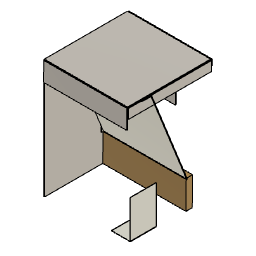
塗装ブース v8 (Autodesk Fusion 360 design; units mm, degrees)
Autodesk Fusion 360 part; units mm, degrees
note: some values were not read from the file. Set by a fixed rule: which face or edge a step refers to.
sketch "スケッチ1" plane through (0, 0, 0) normal (0, 1, 0) x (1, 0, 0) in component "塗装ブース"
  line L0 (0, 0) -> (350, 0)
  line L1 (350, 0) -> (350, -500)
  line L2 (350, -500) -> (0, -500)
  line L3 (0, -500) -> (0, 0)
  line L4 (340, -470) -> (150, -470)
  line L5 (150, -470) -> (150, -280)
  line L6 (150, -280) -> (340, -280)
  line L7 (340, -280) -> (340, -470)
  line L8 (315, -470) -> (315, -500) construction
  line L9 (350, -434.8785) -> (340, -434.8785)
  dimension "d1" = 350
  dimension "d2" = 500
  dimension "d3" = 190
  dimension "d4" = 190
  dimension "d5" = 30
  dimension "d6" = 10
  constraint horizontal L0
  constraint vertical L1
  constraint horizontal L2
  constraint vertical L3
  constraint coincident L0.start L3.end
  constraint horizontal L4
  constraint vertical L5
  constraint horizontal L6
  constraint vertical L7
  constraint coincident L4 L8.start
  constraint coincident L2 L8.end
  constraint perpendicular L2 L8
  constraint coincident L1 L9.start
  constraint coincident L7 L9.end
  constraint perpendicular L7 L9
  measures "d1" distance of L0.start L0.end
  measures "d2" distance of L0.start L2.end
  measures "d3" distance of L4.start L4.end
  measures "d4" distance of L4.start L6.end
  measures "d5" distance of L8.start L8.end
  measures "d6" distance of L9.start L9.end
sketch "スケッチ2" plane through (0, 0, 0) normal (1, 0, 0) x (0, 1, 0) in component "塗装ブース"
  line L0 (0, 0) -> (-350, 0)
  line L1 (-350, 0) -> (-350, 500)
  line L2 (-350, 500) -> (0, 500)
  line L3 (0, 500) -> (0, 0)
  line L4 (0, 500) -> (0, 475)
  line L5 (-205.9711, 100.0797) -> (-180.9711, 100.0797)
  line L6 (-180.9711, 100.0797) -> (-180.9711, 0.0797)
  line L7 (-180.9711, 0.0797) -> (-205.9711, 0.0797)
  line L8 (-205.9711, 0.0797) -> (-205.9711, 100.0797)
  circle A0 centre (0, 475) radius 425 construction
  line L9 (0, 475) -> (-246.3716, 128.6966)
  line L10 (0, 475) -> (-2.4445, 476.7391)
  line L11 (-2.4445, 476.7391) -> (-248.8099, 130.4443)
  line L12 (-246.3716, 128.6966) -> (-248.8099, 130.4443)
  dimension "d7" = 350
  dimension "d8" = 500
  dimension "d9" = 25
  dimension "d10" = 25
  dimension "d11" = 100
  dimension "d12" = 850
  dimension "d13" = 425
  dimension "d14" = 3
  constraint horizontal L0
  constraint vertical L1
  constraint horizontal L2
  constraint vertical L3
  constraint coincident L0.start L3.end
  constraint perpendicular L2 L4
  constraint horizontal L5
  constraint vertical L6
  constraint horizontal L7
  constraint vertical L8
  constraint coincident L4.end A0.centre
  constraint coincident A0 L9.end
  constraint perpendicular L9 L10
  constraint coincident A0 L11.end
  constraint perpendicular L10 L11
  measures "d7" distance of L0.start L0.end
  measures "d8" distance of L0.start L2.end
  measures "d9" distance of L2.end L4.end
  measures "d10" distance of L5.start L5.end
  measures "d11" distance of L5.start L7.end
  measures "d12" diameter of A0
  measures "d13" distance of L4.end L9.end
  measures "d14" distance of L4.end L10.end
extrude "押し出し1" add sketch "スケッチ1" against normal blind 3 makes body 1 in component "塗装ブース"
extrude "押し出し2" add sketch "スケッチ2" along normal blind 3 separate body contours L9 L10 L11 L12 | L0 L1 L2 L3 L4 | L5 L6 L7 L8 makes body 2 in component "塗装ブース"
ref_plane "作業平面1" through (175, -175, 250) normal (-1, 0, 0) x (0, -1, 0) in component "塗装ブース"
mirror "ミラー1" about plane through (175, -175, 250) normal (-1, 0, 0) of bodies 2 makes body 3 in component "塗装ブース"
sketch "スケッチ3" plane through (0, 0, 0) normal (0, 0, 1) x (1, 0, 0) in component "塗装ブース"
  line L0 (0, 0) -> (350, 0)
  line L1 (350, 0) -> (350, -350)
  line L2 (350, -350) -> (0, -350)
  line L3 (0, -350) -> (0, 0)
  dimension "d22" = 350
  dimension "d23" = 350
  constraint horizontal L0
  constraint vertical L1
  constraint horizontal L2
  constraint vertical L3
  constraint coincident L0.start L3.end
  measures "d22" distance of L0.start L0.end
  measures "d23" distance of L0.start L2.end
extrude "押し出し3" add sketch "スケッチ3" along normal blind 3 separate body makes body 4 in component "塗装ブース"
extrude "押し出し4" add sketch "スケッチ2" along normal blind 350 separate body contours L9 L10 L11 L12 makes body 5 in component "塗装ブース"
extrude "押し出し5" add sketch "スケッチ2" along normal blind 350 separate body contours L5 L6 L7 L8 makes body 6 in component "塗装ブース"
move_body "移動1" bodies 5 to x (1, 0, 0) y (0, 0.992546, 0.121869) z (0, -0.121869, 0.992546) at (0, 58.0817, 3.8514) in component "塗装ブース"
move_face "面を移動1" by (5, 0, 0) 1 faces at (0, -135.5716, 226.6252) on bodies 5 in component "塗装ブース"
move_face "面を移動2" by (-5, 0, 0) 1 faces at (350, -135.5716, 226.6252) on bodies 5 in component "塗装ブース"
copy_body "ボディのコピーと貼り付け1" bodies 4 makes body 7 in component "塗装ブース"
move_body "移動2" bodies 7 to x (1, 0, 0) y (0, 1, 0) z (0, 0, 1) at (0, 0, 500) in component "塗装ブース"
sketch "スケッチ4" plane through (3, 0, 0) normal (1, 0, 0) x (0, 1, 0) in component "塗装ブース"
  line L0 (0, 500) -> (-350, 500)
  line L1 (-350, 500) -> (-350, 0)
  line L2 (-350, 0) -> (0, 0)
  line L3 (0, 0) -> (0, 500)
  line L4 (0, 200) -> (-100, 0)
  line L5 (-100, 0) -> (-102.6833, 1.3416)
  line L6 (0, 200) -> (-2.6833, 201.3416)
  line L7 (-2.6833, 201.3416) -> (-102.6833, 1.3416)
  dimension "d30" = 3
  dimension "d31" = 3
  constraint coincident L3 L4.start
  constraint coincident L2 L4.end
  constraint perpendicular L4 L5
  constraint perpendicular L4 L6
  measures "d30" distance of L4.end L5.end
  measures "d31" distance of L4.start L6.end
extrude "押し出し6" add sketch "スケッチ4" along normal blind 340 separate body contours L4 L5 L6 L7 makes body 8 in component "塗装ブース"
move_body "移動3" bodies 8 to x (1, 0, 0) y (0, 1, 0) z (0, 0, 1) at (0, 0, 75) in component "塗装ブース"
move_face "面を移動3" by (0, -36.6715, -73.343) 1 faces at (116.3333, -100.8944, 75.4472) on bodies 8 in component "塗装ブース"
move_face "面を移動4" by (0, -40.2492, -80.4984) 1 faces at (229.6667, -1.7889, 275.8944) on bodies 8 in component "塗装ブース"
move_body "移動4" bodies 8 to x (1, 0, 0) y (0, 1, 0) z (0, 0, 1) at (0, 41, 0) in component "塗装ブース"
move_body "移動5" bodies 5 to x (1, 0, 0) y (0, 0.642788, 0.766044) z (0, -0.766044, 0.642788) at (0, 5.7568, 193.6568) in component "塗装ブース"
move_body "移動6" bodies 5 to x (1, 0, 0) y (0, 1, 0) z (0, 0, 1) at (0, 100, 0) in component "塗装ブース"
move_body "移動7" bodies 6 to x (1, 0, 0) y (0, 1, 0) z (0, 0, 1) at (0, 100, 0) in component "塗装ブース"
move_body "移動8" bodies 5 to x (1, 0, 0) y (0, 0.984808, 0.173648) z (0, -0.173648, 0.984808) at (0, 16.2943, 19.7581) in component "塗装ブース"
move_body "移動9" bodies 5 to x (1, 0, 0) y (0, 0.996195, -0.087156) z (0, 0.087156, 0.996195) at (0, -2.7934, -12.609) in component "塗装ブース"
move_face "面を移動5" by (0, 26.8381, -53.663) 1 faces at (118.3333, -286.4983, 480.1295) on bodies 5 in component "塗装ブース"
copy_body "ボディのコピーと貼り付け2" bodies 5 makes body 9 in component "塗装ブース"
move_body "移動10" bodies 9 to x (1, 0, 0) y (0, 0.891007, -0.45399) z (0, 0.45399, 0.891007) at (0, -231.01, -96.0407) in component "塗装ブース"
move_face "面を移動6" by (0, -2.0979, -279.9921) 1 faces at (118.3333, -268.7571, 401.827) on bodies 9 in component "塗装ブース"
move_body "移動11" bodies 9 to x (1, 0, 0) y (0, 1, 0) z (0, 0, 1) at (0, -25.6328, 378.6324) in component "塗装ブース"
move_face "面を移動7" by (0, -0.2755, -24.9985) 1 faces at (118.3333, -297.1247, 415.4732) on bodies 9 in component "塗装ブース"
copy_body "ボディのコピーと貼り付け3" bodies 6 makes body 10 in component "塗装ブース"
move_body "移動12" bodies 10 to x (1, 0, 0) y (0, 1, 0) z (0, 0, 1) at (0, 60, 0) in component "塗装ブース"
move_body "位置合わせ1" bodies 10 to x (1, 0, 0) y (0, 0.894383, 0.447302) z (0, -0.447302, 0.894383) at (0, 0.4446, 11.3952) in component "塗装ブース"
move_body "移動13" bodies 10 to x (1, 0, 0) y (0, 1, 0) z (0, 0, 1) at (0, -8.946, 17.8877) in component "塗装ブース"
copy_body "ボディのコピーと貼り付け4" bodies 10 makes body 11 in component "塗装ブース"
move_body "移動14" bodies 11 to x (1, 0, 0) y (0, 1, 0) z (0, 0, 1) at (0, -190.1033, 380.1128) in component "塗装ブース"
move_face "面を移動8" by (0, 17.8921, -35.7753) 1 faces at (118.3333, -259.6601, 426.4665) on bodies 5 in component "塗装ブース"
copy_body "ボディ -> コンポーネント1" bodies 5 removing the originals makes body 12 in component "中板1"
copy_body "CutPasteBodies1" bodies 11 10 removing the originals makes body 13 makes body 14 in component "中板1"
move_body "移動1'" bodies 13 to x (1, 0, 0) y (0, 1, 0) z (0, 0, 1) at (0, -4.473, 8.9438) in component "中板1"
move_face "面を移動1'" by (0, -6.2622, 12.5214) 1 faces at (118.3333, -241.7681, 390.6912) on bodies 12 in component "中板1"
copy_body "CutPasteBodies5" bodies 13 14 removing the originals makes body 15 makes body 16 in component "塗装ブース"
move_body "移動15" bodies 16 to x (1, 0, 0) y (0, 0.891007, -0.45399) z (0, 0.45399, 0.891007) at (0, -55.0194, -27.1445) in component "塗装ブース"
move_body "移動16" bodies 15 to x (1, 0, 0) y (0, 0.898794, -0.438371) z (0, 0.438371, 0.898794) at (0, -245.4958, -66.4217) in component "塗装ブース"
move_body "移動17" bodies 15 to x (1, 0, 0) y (0, 1, 0) z (0, 0, 1) at (0, 49.9975, 0.498) in component "塗装ブース"
move_body "移動18" bodies 16 to x (1, 0, 0) y (0, 1, 0) z (0, 0, 1) at (0, -29.9992, 0.2248) in component "塗装ブース"
move_body "移動2'" bodies 12 to x (1, 0, 0) y (0, 0.996195, -0.087156) z (0, 0.087156, 0.996195) at (0, -36.015, -20.2422) in component "中板1"
move_face "面を移動2'" by (0, -4.3724, 11.1751) 1 faces at (118.3333, -123.3274, 87.7986) on bodies 12 in component "中板1"
move_face "面を移動9" by (0, 0.5511, 49.997) 1 faces at (118.3333, -297.312, 390.4737) on bodies 9 in component "塗装ブース"
move_face "面を移動3'" by (0, -11.0295, 27.8989) 1 faces at (118.3333, -247.9591, 403.0533) on bodies 12 in component "中板1"
move_body "移動3'" bodies 12 to x (1, 0, 0) y (0, 0.996195, -0.087156) z (0, 0.087156, 0.996195) at (0, -9.0544, -10.9217) in component "中板1"
move_body "移動19" bodies 9 to x (1, 0, 0) y (0, 1, 0) z (0, 0, 1) at (0, 39.9989, -0.2997) in component "塗装ブース"
move_body "移動4'" bodies 12 to x (1, 0, 0) y (0, 1, 0) z (0, 0, 1) at (0, -2.852, 9.5847) in component "中板1"
move_body "移動20" bodies 9 to x (1, 0, 0) y (0, 1, 0) z (0, 0, 1) at (0, -19.9994, 0.1498) in component "塗装ブース"
move_face "面を移動4'" by (0, 2.8181, -9.5947) 1 faces at (118.3333, -130.5347, 108.3778) on bodies 12 in component "中板1"
move_body "移動5'" bodies 12 to x (1, 0, 0) y (0, 0.996195, 0.087156) z (0, -0.087156, 0.996195) at (0, 8.0681, 11.6693) in component "中板1"
move_body "移動21" bodies 9 to x (1, 0, 0) y (0, 1, 0) z (0, 0, 1) at (0, -73.9979, 0.5544) in component "塗装ブース"
move_face "面を移動5'" by (0, -7.353, 18.5993) 1 faces at (118.3333, -262.6651, 440.2519) on bodies 12 in component "中板1"
move_face "面を移動10" by (0, -0.2204, -19.9988) 1 faces at (118.3333, -350.9359, 440.8772) on bodies 9 in component "塗装ブース"
sketch "スケッチ5" plane through (3, 0, 0) normal (1, 0, 0) x (0, 1, 0) in component "塗装ブース"
  line L0 (0, 500) -> (-350, 500)
  line L1 (-350, 500) -> (-350, 0)
  line L2 (-350, 0) -> (0, 0)
  line L3 (0, 0) -> (0, 500)
  line L4 (-350, 500) -> (-240, 500)
  line L5 (-240, 500) -> (-240, 460)
  line L6 (-240, 460) -> (-350, 460)
  line L7 (-350, 460) -> (-350, 500)
  line L8 (-350, 0) -> (-100, 0)
  line L9 (-100, 0) -> (-100, 120)
  line L10 (-100, 120) -> (-350, 120)
  line L11 (-350, 120) -> (-350, 0)
  line L12 (-100, 120) -> (-73, 120)
  line L13 (-73, 120) -> (-73, 0)
  line L14 (-73, 0) -> (-100, 0)
  line L15 (-100, 0) -> (-100, 120)
  line L16 (-240, 460) -> (-99.0891, 105.2934)
  line L17 (-99.0891, 105.2934) -> (-96.3011, 106.4009)
  line L18 (-240, 460) -> (-237.2119, 461.1076)
  line L19 (-237.2119, 461.1076) -> (-96.3011, 106.4009)
  dimension "d46" = 250
  dimension "d47" = 120
  dimension "d48" = 40
  dimension "d49" = 110
  dimension "d50" = 27
  dimension "d51" = 120
  dimension "d52" = 3
  dimension "d53" = 3
  constraint horizontal L4
  constraint vertical L5
  constraint horizontal L6
  constraint vertical L7
  constraint coincident L0.end L1.start
  constraint horizontal L8
  constraint vertical L9
  constraint horizontal L10
  constraint vertical L11
  constraint coincident L1.end L2.start
  constraint horizontal L12
  constraint vertical L13
  constraint horizontal L14
  constraint vertical L15
  constraint perpendicular L16 L17
  constraint perpendicular L16 L18
  constraint perpendicular L17 L19
  measures "d46" distance of L1.end L8.end
  measures "d47" distance of L1.end L10.end
  measures "d48" distance of L4.end L5.end
  measures "d49" distance of L5.end L6.end
  measures "d50" distance of L9.end L12.end
  measures "d51" distance of L9.end L8.end
  measures "d52" distance of L16.end L17.end
  measures "d53" distance of L5.end L18.end
extrude "押し出し7" add sketch "スケッチ5" along normal blind 340 separate body contours L10 L16 L18 L19 makes body 17 in component "塗装ブース"
move_face "面を移動11" by (0, 1.9999, -0.015) 1 faces at (116.6667, -99.7697, 69.9327) on bodies 16 in component "塗装ブース"
move_face "面を移動12" by (0, 0.1498, 19.9994) 1 faces at (116.6667, -115.5195, 103.385) on bodies 16 in component "塗装ブース"
move_body "移動22" bodies 16 to x (1, 0, 0) y (0, 1, 0) z (0, 0, 1) at (0, -8.7841, -3.4099) in component "塗装ブース"
move_body "移動23" bodies 16 to x (1, 0, 0) y (0, 1, 0) z (0, 0, 1) at (0, 29.9992, -0.2248) in component "塗装ブース"
copy_body "ボディのコピーと貼り付け6" bodies 9 makes body 18 in component "塗装ブース"
move_body "移動24" bodies 18 to x (1, 0, 0) y (0, 1, 0) z (0, 0, 1) at (0, 249.993, -1.8731) in component "塗装ブース"
sketch "スケッチ6" plane through (3, 0, 0) normal (1, 0, 0) x (0, 1, 0) in component "塗装ブース"
  circle A0 centre (-110, 130) radius 4
  line L0 (-350, 0) -> (-110, 0)
  line L1 (-110, 0) -> (-110, 130)
  line L2 (-110, 130) -> (-350, 130)
  line L3 (-350, 130) -> (-350, 0)
  line L4 (-350, 500) -> (-245, 500)
  line L5 (-245, 500) -> (-245, 464)
  line L6 (-245, 460) -> (-350, 460)
  line L7 (-350, 460) -> (-350, 500)
  line L8 (-246.9279, 456.4953) -> (-248.453, 453.7226)
  line L9 (-241.5481, 462.0211) -> (-238.8174, 463.6199)
  line L10 (-231.7545, 450.441) -> (-229.1103, 451.8581)
  line L11 (-229.1103, 451.8581) -> (-236.9376, 466.4634)
  line L12 (-236.9376, 466.4634) -> (-244.3537, 467.1352)
  line L13 (-237.1247, 460.4616) -> (-239.7689, 459.0445)
  line L14 (-239.7689, 459.0445) -> (-234.451, 449.1215)
  line L15 (-234.451, 449.1215) -> (-237.0952, 447.7044)
  line L16 (-237.0952, 447.7044) -> (-240.6869, 454.4064)
  line L17 (-240.6869, 454.4064) -> (-239.7689, 459.0445)
  line L18 (-239.7689, 459.0445) -> (-241.5665, 462.0521)
  arc A1 (-241.5481, 462.0211) -> (-246.9279, 456.4953) centre (-245, 460) ccw
  line L19 (-238.8174, 463.6199) -> (-238.5621, 463.1437)
  line L20 (-237.1247, 460.4616) -> (-231.7545, 450.441)
  arc A2 (-238.5621, 463.1437) -> (-238.8174, 463.6199) centre (-245, 460) ccw
  arc A3 (-244.3537, 467.1352) -> (-248.453, 453.7226) centre (-245, 460) ccw
  circle A4 centre (-245, 460) radius 4
  dimension "d57" = 8
  dimension "d58" = 240
  dimension "d59" = 130
  dimension "d60" = 8
  dimension "d61" = 105
  dimension "d62" = 40
  dimension "d63" = 3
  dimension "d64" = 3
  dimension "d65" = 3
  dimension "d66" = 8
  constraint horizontal L0
  constraint vertical L1
  constraint horizontal L2
  constraint vertical L3
  constraint coincident A0.centre L1.end
  constraint horizontal L4
  constraint vertical L5
  constraint horizontal L6
  constraint vertical L7
  constraint coincident L6.start A1.centre
  constraint concentric A1 A2
  constraint perpendicular L10 L19
  constraint perpendicular L10 L11
  constraint coincident L12.end A2
  constraint tangent L12 A2
  constraint coincident L13.start L19
  constraint perpendicular L13 L19
  constraint perpendicular L13 L14
  constraint perpendicular L14 L15
  constraint perpendicular L15 L16
  constraint coincident L18.end A1
  constraint tangent L18 A1
  constraint collinear L19 L20
  constraint concentric A2 A3
  constraint coincident A1 L5.end
  measures "d57" diameter of A0
  measures "d58" distance of L0.start L0.end
  measures "d59" distance of L0.start L2.end
  measures "d60" diameter of A1
  measures "d61" distance of L4.start L4.end
  measures "d62" distance of L4.end L6.start
  measures "d63" distance of L10.start L10.end
  measures "d64" distance of L13.start L13.end
  measures "d65" distance of L14.end L15.end
  measures "d66" diameter of A4
move_face "面を移動13" by (0, -0.5511, -49.997) 1 faces at (118.3333, -101.0927, 419.0045) on bodies 18 in component "塗装ブース"
move_body "移動25" bodies 18 to x (1, 0, 0) y (0, 1, 0) z (0, 0, 1) at (0, -24.9993, 0.1873) in component "塗装ブース"
extrude "押し出し1'" add sketch "スケッチ6" along normal blind 370 and the other way blind 20 separate body contours L18 A1 A4 makes body 19
copy_body "CutPasteBodies7" bodies 19 removing the originals makes body 20 in component "塗装ブース"
copy_body "ボディのコピーと貼り付け1'" bodies 20 makes body 21
move_body "移動1''" bodies 21 to x (1, 0, 0) y (0, 1, 0) z (0, 0, 1) at (0, 117.9673, -299.029)
copy_body "ボディのコピーと貼り付け2'" bodies 20 makes body 22
move_body "移動2''" bodies 22 to x (1, 0, 0) y (0, 1, 0) z (0, 0, 1) at (0, 112, -84)
move_body "移動26" bodies 20 to x (1, 0, 0) y (0, 1, 0) z (0, 0, 1) at (0, 0, 25) in component "塗装ブース"
move_body "移動27" bodies 20 to x (1, 0, 0) y (0, 1, 0) z (0, 0, 1) at (0, 0, -20) in component "塗装ブース"
move_body "移動3''" bodies 22 to x (1, 0, 0) y (0, 1, 0) z (0, 0, 1) at (0, 12, 13)
sketch "スケッチ1 (2)" plane through (3, 0, 0) normal (1, 0, 0) x (0, 1, 0)
  line L0 (-275, 0) -> (-165, 0)
  line L1 (-165, 0) -> (-165, 1)
  line L2 (-165, 1) -> (-275, 1)
  line L3 (-275, 1) -> (-275, 0)
  dimension "d83" = 110
  dimension "d84" = 1
  constraint horizontal L0
  constraint vertical L1
  constraint horizontal L2
  constraint vertical L3
  measures "d83" distance of L0.start L0.end
  measures "d84" distance of L0.start L2.end
extrude "押し出し2'" add sketch "スケッチ1 (2)" along normal blind 80 separate body makes body 23
sketch "スケッチ2 (2)" plane through (0, 0, 1) normal (0, 0, 1) x (-1, 0, 0)
  line L0 (-3, 165) -> (-3, 275)
  line L1 (-3, 275) -> (-83, 275)
  line L2 (-83, 275) -> (-83, 165)
  line L3 (-83, 165) -> (-3, 165)
  line L4 (-3, 165) -> (-4, 165)
  line L5 (-4, 165) -> (-4, 275)
  line L6 (-4, 275) -> (-3, 275)
  line L7 (-3, 275) -> (-3, 165)
  dimension "d87" = 1
  dimension "d88" = 110
  constraint horizontal L4
  constraint vertical L5
  constraint horizontal L6
  constraint vertical L7
  constraint coincident L0.start L3.end
  measures "d87" distance of L0.start L4.end
  measures "d88" distance of L0.start L0.end
extrude "押し出し3'" add sketch "スケッチ2 (2)" along normal blind 160 contours L0 L1 L3 L4 L5 L6 L7 bodies 23
move_body "移動4''" bodies 23 to x (1, 0, 0) y (0, 1, 0) z (0, 0, 1) at (10, 0, 10)
move_body "移動5''" bodies 23 to x (1, 0, 0) y (0, 1, 0) z (0, 0, 1) at (0, 0, -7)
move_body "移動6'" bodies 23 to x (1, 0, 0) y (0, 1, 0) z (0, 0, 1) at (-10, 0, 0)
move_body "移動7'" bodies 23 to x (1, 0, 0) y (0, 1, 0) z (0, 0, 1) at (0, 20, 0)
ref_plane "作業平面1" through (175, -175, 250) normal (-1, 0, 0) x (0, 0, -1)
mirror "ミラー1'" about plane through (175, -175, 250) normal (-1, 0, 0) of bodies 23 makes body 24
copy_body "CutPasteBodies8" bodies 21 22 23 24 removing the originals makes body 25 makes body 26 makes body 27 makes body 28 in component "塗装ブース"
delete_body "RemoveBody5" bodies 8 in component "塗装ブース"
delete_body "RemoveBody6" bodies 6 in component "塗装ブース"
move_body "移動28" bodies 18 26 to x (1, 0, 0) y (0, 1, 0) z (0, 0, 1) at (0, -20, 0) in component "塗装ブース"
move_body "移動29" bodies 27 28 to x (1, 0, 0) y (0, 1, 0) z (0, 0, 1) at (0, -80, 0) in component "塗装ブース"
copy_body "ボディのコピーと貼り付け1''" bodies 1 2 4 3 7 9 16 20 15 25 18 27 28 17 26 makes body 29 makes body 30 makes body 31 makes body 32 makes body 33 makes body 34 makes body 35 makes body 36 makes body 37 makes body 38 makes body 39 makes body 40 makes body 41 makes body 42 makes body 43 in component "塗装ブース2"
sketch "スケッチ1 (3)" plane through (0, 0, 3) normal (0, 0, 1) x (-1, 0, 0) in component "塗装ブース2"
  line L0 (0, 350) -> (-350, 350)
  line L1 (-350, 350) -> (-350, 0)
  line L2 (-350, 0) -> (0, 0)
  line L3 (0, 0) -> (0, 350)
  line L4 (-38.9588, 123.5058) -> (-158.9588, 123.5058)
  line L5 (-158.9588, 123.5058) -> (-158.9588, 150.5058)
  line L6 (-158.9588, 150.5058) -> (-38.9588, 150.5058)
  line L7 (-38.9588, 150.5058) -> (-38.9588, 123.5058)
  dimension "d111" = 120
  dimension "d112" = 27
  constraint horizontal L4
  constraint vertical L5
  constraint horizontal L6
  constraint vertical L7
  measures "d111" distance of L4.start L4.end
  measures "d112" distance of L4.start L6.end
extrude "押し出し1''" add sketch "スケッチ1 (3)" along normal blind 485 separate body contours L4 L5 L6 L7 makes body 44 in component "塗装ブース2"
copy_body "ボディのコピーと貼り付け2''" bodies 44 makes body 45 in component "塗装ブース2"
move_body "移動1'''" bodies 45 to x (1, 0, 0) y (0, 1, 0) z (0, 0, 1) at (120, 0, 0) in component "塗装ブース2"
move_body "移動2'''" bodies 44 45 to x (1, 0, 0) y (0, 1, 0) z (0, 0, 1) at (-35, 0, 0) in component "塗装ブース2"
delete_body "RemoveBody7" bodies 15 in component "塗装ブース"
move_face "面を移動14" by (0, -14.7678, 37.1741) 1 faces at (116.3333, -239.0706, 460.3692) on bodies 17 in component "塗装ブース"
sketch "スケッチ7" plane through (0, -49.4554, -19.6467) normal (0, -0.929352, -0.369195) x (1, 0, 0) in component "塗装ブース"
  line L0 (3, 556.1087) -> (3, 150.2624)
  line L1 (3, 150.2624) -> (343, 150.2624)
  line L2 (343, 150.2624) -> (343, 556.1087)
  line L3 (343, 556.1087) -> (3, 556.1087)
  line L4 (3, 556.1087) -> (18, 556.1087)
  line L5 (18, 556.1087) -> (18, 546.1087)
  line L6 (18, 546.1087) -> (3, 546.1087)
  line L7 (3, 546.1087) -> (3, 556.1087)
  line L8 (343, 556.1087) -> (328, 556.1087)
  line L9 (328, 556.1087) -> (328, 546.1087)
  line L10 (328, 546.1087) -> (343, 546.1087)
  line L11 (343, 546.1087) -> (343, 556.1087)
  line L12 (18, 546.1087) -> (328.5453, 546.1087)
  line L13 (328.5453, 546.1087) -> (328.5453, 506.1087)
  line L14 (328.5453, 506.1087) -> (18, 506.1087)
  line L15 (18, 506.1087) -> (18, 546.1087)
  dimension "d115" = 15
  dimension "d116" = 10
  dimension "d117" = 15
  dimension "d118" = 10
  dimension "d119" = 310.5453
  dimension "d120" = 40
  constraint horizontal L4
  constraint vertical L5
  constraint horizontal L6
  constraint vertical L7
  constraint coincident L0.start L3.end
  constraint horizontal L8
  constraint vertical L9
  constraint horizontal L10
  constraint vertical L11
  constraint coincident L2.end L3.start
  constraint horizontal L12
  constraint vertical L13
  constraint horizontal L14
  constraint vertical L15
  measures "d115" distance of L0.start L4.end
  measures "d116" distance of L0.start L6.end
  measures "d117" distance of L2.end L8.end
  measures "d118" distance of L2.end L10.end
  measures "d119" distance of L5.end L12.end
  measures "d120" distance of L5.end L14.end
extrude "押し出し8" cut sketch "スケッチ7" against normal blind 20 contours L10 L12 L13 L14 L15 bodies 17 in component "塗装ブース"
move_face "面を移動15" by (0, 0.4409, 39.9976) 1 faces at (118.3333, -146.4667, 369.193) on bodies 18 in component "塗装ブース"
copy_body "ボディのコピーと貼り付け9" bodies 9 makes body 46 in component "塗装ブース"
move_body "移動30" bodies 46 to x (1, 0, 0) y (0, 0, -1) z (0, 1, 0) at (0, -715.392, 145.3667) in component "塗装ブース"
move_face "面を移動16" by (0, -39.9989, 0.2997) 1 faces at (118.3333, -214.5202, 495.853) on bodies 46 in component "塗装ブース"
move_face "面を移動17" by (0, -3.6919, 9.2935) 1 faces at (225.0302, -235.3787, 451.0757) on bodies 17 in component "塗装ブース"
sketch "スケッチ8" plane through (3, 0, 0) normal (1, 0, 0) x (0, 1, 0) in component "塗装ブース"
extrude "押し出し9" add sketch "スケッチ5" along normal blind 340 contours L9 L10 L15 L16 L19 | L9 L15 L16 L17 L19 bodies 17 in component "塗装ブース"
move_face "面を移動18" by (10, 0, 0) 1 faces at (343, -149.1233, 236.6587) on bodies 17 in component "塗装ブース"
move_body "移動31" bodies 2 to x (1, 0, 0) y (0, 1, 0) z (0, 0, 1) at (-3, 0, 0) in component "塗装ブース"
move_body "移動32" bodies 3 to x (1, 0, 0) y (0, 1, 0) z (0, 0, 1) at (3, 0, 0) in component "塗装ブース"
move_body "移動33" bodies 1 to x (1, 0, 0) y (0, 1, 0) z (0, 0, 1) at (0, 3, 0) in component "塗装ブース"
move_body "移動34" bodies 4 to x (1, 0, 0) y (0, 1, 0) z (0, 0, 1) at (0, 0, -3) in component "塗装ブース"
move_body "移動35" bodies 9 to x (1, 0, 0) y (0, 1, 0) z (0, 0, 1) at (-5.0412, 3.6759, -1.0303) in component "塗装ブース"
move_face "面を移動19" by (10, 0, 0) 1 faces at (339.9588, -347.21, 446.5132) on bodies 9 in component "塗装ブース"
move_body "移動36" bodies 9 to x (1, 0, 0) y (0, 1, 0) z (0, 0, 1) at (0, -3.9999, 0.03) in component "塗装ブース"
move_face "面を移動20" by (0, 28.9186, -72.7952) 1 faces at (119.6667, -98.1598, 105.6625) on bodies 17 in component "塗装ブース"
move_face "面を移動21" by (0, -33.2275, 83.6417) 1 faces at (119.6667, -69.2411, 32.8673) on bodies 17 in component "塗装ブース"
move_body "移動37" bodies 46 to x (1, 0, 0) y (0, 1, 0) z (0, 0, 1) at (-2, 0, 0) in component "塗装ブース"
move_face "面を移動22" by (10, 0, 0) 1 faces at (343, -281.1814, 496.3525) on bodies 46 in component "塗装ブース"
move_face "面を移動23" by (9.455, 0, 0) 1 faces at (328.5453, -246.4545, 478.9562) on bodies 17 in component "塗装ブース"
move_face "面を移動24" by (10, 0, 0) 1 faces at (345, -145.9422, 439.1912) on bodies 18 in component "塗装ブース"
copy_body "CutPasteBodies1'" bodies 2 7 9 18 removing the originals makes body 47 makes body 48 makes body 49 makes body 50 in component "001"
copy_body "CutPasteBodies1''" bodies 1 4 3 removing the originals makes body 51 makes body 52 makes body 53 in component "002"
move_body "移動1''''" bodies 50 to x (1, 0, 0) y (0, 1, 0) z (0, 0, 1) at (-5, 0, 0) in component "001"
copy_body "CutPasteBodies1'''" bodies 46 17 removing the originals makes body 54 makes body 55 in component "003"
delete_body "RemoveBody17" bodies 17 in component "塗装ブース"
delete_body "RemoveBody18" bodies 46 in component "塗装ブース"
sketch "スケッチ9" plane through (0, 0, 0) normal (1, 0, 0) x (0, 1, 0) in component "塗装ブース"
  line L0 (0, 500) -> (-350, 500)
  line L1 (-350, 500) -> (-350, 0)
  line L2 (-350, 0) -> (0, 0)
  line L3 (0, 0) -> (0, 500)
  line L4 (-90, 110) -> (-106, 110)
  line L5 (-106, 110) -> (-106, 182)
  line L6 (-106, 182) -> (-90, 182)
  line L7 (-90, 182) -> (-90, 110)
  line L8 (-90, 110) -> (-106, 182) construction
  line L9 (-106, 110) -> (-90, 182) construction
  line L10 (0, 150) -> (-90, 150)
  line L11 (-90, 0) -> (-90, 110)
  point P0 (-98, 146)
  dimension "d125" = 16
  dimension "d126" = 72
  dimension "d127" = 90
  dimension "d128" = 110
  constraint horizontal L4
  constraint perpendicular L4 L5
  constraint parallel L4 L6
  constraint parallel L5 L7
  constraint coincident L8 P0
  constraint coincident L9 P0
  constraint coincident L3 L10.start
  constraint perpendicular L7 L10
  constraint coincident L2 L11.start
  constraint perpendicular L4 L11
  measures "d125" distance of L5.end L6.end
  measures "d126" distance of L4.end L5.end
  measures "d127" distance of L10.start L10.end
  measures "d128" distance of L11.start L4.start
extrude "押し出し10" add sketch "スケッチ9" along normal blind 2 separate body contours L4 L5 L6 L7 makes body 56 in component "塗装ブース"
copy_body "ボディのコピーと貼り付け10" bodies 50 makes body 57 in component "塗装ブース"
move_body "移動38" bodies 57 to x (1, 0, 0) y (0, 1, 0) z (0, 0, 1) at (0, 151.0107, 0.8686) in component "塗装ブース"
move_face "面を移動25" by (0, 0.5511, 49.997) 1 faces at (116.6667, 4.8438, 410.0607) on bodies 57 in component "塗装ブース"
copy_body "CutPasteBodies2" bodies 57 removing the originals makes body 58 in component "001"
copy_body "ボディのコピーと貼り付け2'''" bodies 52 makes body 59 in component "002"
move_body "移動1'''''" bodies 59 to x (1, 0, 0) y (0, 1, 0) z (0, 0, 1) at (-400, 0, 0) in component "002"
move_face "面を移動1''" by (310, 0, 0) 1 faces at (-400, -233.3333, -1) on bodies 59 in component "002"
move_body "移動2''''" bodies 59 to x (0, 0, -1) y (0, 1, 0) z (1, 0, 0) at (-2, 0, -53) in component "002"
copy_body "ボディのコピーと貼り付け3'" bodies 59 makes body 60 in component "001"
move_body "移動2'''''" bodies 60 to x (1, 0, 0) y (0, 1, 0) z (0, 0, 1) at (356, 0, 463) in component "001"
copy_body "ボディのコピーと貼り付け3''" bodies 51 makes body 61 in component "002"
move_body "移動3'''" bodies 61 to x (1, 0, 0) y (0, 1, 0) z (0, 0, 1) at (-425, 0, 0) in component "002"
move_face "面を移動2''" by (-310, 0, 0) 2 faces at (-75, 1, 144.9595) (-75, 2, 456.5857) on bodies 61 in component "002"
move_body "移動4'''" bodies 61 to x (1, 0, 0) y (0, 1, 0) z (0, 0, 1) at (380, 0, 0) in component "002"
move_body "移動5'''" bodies 61 to x (0, 1, 0) y (-1, 0, 0) z (0, 0, 1) at (-2, 8, 0) in component "002"
move_face "面を移動3''" by (0, -50, 0) 1 faces at (-4, 0, 23.6667) on bodies 59 in component "002"
copy_body "ボディのコピーと貼り付け11" bodies 52 makes body 62 in component "塗装ブース"
move_body "移動39" bodies 62 to x (1, 0, 0) y (0, 1, 0) z (0, 0, 1) at (0, 390, 0) in component "塗装ブース"
move_face "面を移動26" by (0, -310, 0) 1 faces at (116.6667, 390, -1) on bodies 62 in component "塗装ブース"
move_body "移動40" bodies 62 to x (1, 0, 0) y (0, 1, 0) z (0, 0, 1) at (0, -35, 0) in component "塗装ブース"
move_body "移動41" bodies 62 to x (1, 0, 0) y (0, 0, 1) z (0, -1, 0) at (0, 2, -8) in component "塗装ブース"
copy_body "CutPasteBodies4" bodies 62 removing the originals makes body 63 in component "002"
move_face "面を移動1'''" by (0, 0.1653, 14.9991) 1 faces at (116.6667, 5.2184, 460.0596) on bodies 58 in component "001"
move_body "移動42" bodies 56 to x (1, 0, 0) y (0, 0, 1) z (0, -1, 0) at (0, 40, 224) in component "塗装ブース"
move_body "移動43" bodies 56 to x (1, 0, 0) y (0, 1, 0) z (0, 0, 1) at (0, 20, 0) in component "塗装ブース"
copy_body "ボディのコピーと貼り付け12" bodies 56 makes body 64 in component "塗装ブース"
move_body "移動44" bodies 64 to x (1, 0, 0) y (0, 1, 0) z (0, 0, 1) at (350, 0, 0) in component "塗装ブース"
copy_body "CutPasteBodies5'" bodies 64 removing the originals makes body 65 in component "002"
copy_body "CutPasteBodies4'" bodies 56 removing the originals makes body 66 in component "001"
delete_body "RemoveBody23" bodies 20 in component "塗装ブース"
delete_body "RemoveBody24" bodies 25 in component "塗装ブース"
delete_body "RemoveBody25" bodies 26 in component "塗装ブース"
move_body "移動3''''" bodies 66 to x (1, 0, 0) y (0, 1, 0) z (0, 0, 1) at (0, 15, 0) in component "001"
move_body "移動6''" bodies 65 to x (1, 0, 0) y (0, 1, 0) z (0, 0, 1) at (0, 15, 0) in component "002"
move_body "移動7''" bodies 65 to x (1, 0, 0) y (0, 1, 0) z (0, 0, 1) at (0, -5, 0) in component "002"
move_body "移動4''''" bodies 66 to x (1, 0, 0) y (0, 1, 0) z (0, 0, 1) at (0, -5, 0) in component "001"
component "塗装ブース" placed x (1, 0, 0) y (0, 1, 0) z (0, 0, 1) at (0, 0, 0)
component "塗装ブース2" placed x (1, 0, 0) y (0, 1, 0) z (0, 0, 1) at (0, 0, 0)
component "001" placed x (1, 0, 0) y (0, 1, 0) z (0, 0, 1) at (0, 0, 0) in component "塗装ブース"
component "002" placed x (1, 0, 0) y (0, 1, 0) z (0, 0, 1) at (0, 0, 0) in component "塗装ブース"
component "003" placed x (1, 0, 0) y (0, 1, 0) z (0, 0, 1) at (0, 0, 0) in component "塗装ブース"
hidden bodies 27 32 33 34 35 36 37 38 39 42 43
named bodies: "中板1", "爪とぎ", "中板2", "正面", "爪とぎ (1)", "爪とぎ (1) (1)", "爪とぎ (1) (2)", "仲板Main", "中板1 (1)", "仕切り板", "8mm棒1", "8mm棒2", "8mm棒3", "ブックスタンド1", "ブックスタンド2", "中板1 (2)", "仕切り板 (1)", "下 (1)", "奥 (1)", "下 (1) (1)"
